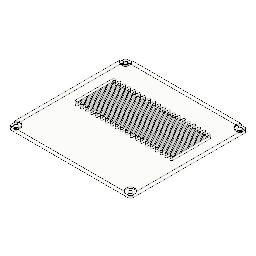
CaseLid v4 (Autodesk Fusion 360 design; units mm, degrees)
Autodesk Fusion 360 part; units mm, degrees
sketch "Sketch1" plane through (0, 0, 0) normal (0, 0, 1) x (1, 0, 0)
  line L0 (0, 0) -> (98, 0)
  line L1 (98, 0) -> (98, 94)
  line L2 (98, 94) -> (0, 94)
  line L3 (0, 94) -> (0, 0)
  dimension "d1" = 98
  dimension "d2" = 94
  constraint horizontal L0
  constraint vertical L1
  constraint horizontal L2
  constraint vertical L3
  constraint coincident L0.start L3.end
  measures "d1" distance of L0.start L0.end
  measures "d2" distance of L0.start L2.end
extrude "Extrude1" add sketch "Sketch1" along normal blind 3
fillet "Fillet1" radius 2 4 edges at (98, 0, 1.5) (98, 94, 1.5) (0, 94, 1.5) (0, 0, 1.5)
sketch "Sketch2" plane through (0, 0, 3) normal (0, 0, 1) x (-1, 0, 0)
  arc A0 (0, -2) -> (-2, 0) centre (-2, -2) ccw
  line L0 (-2, 0) -> (-96, 0)
  arc A1 (-96, 0) -> (-98, -2) centre (-96, -2) ccw
  line L1 (-98, -2) -> (-98, -92)
  arc A2 (-98, -92) -> (-96, -94) centre (-96, -92) ccw
  line L2 (-96, -94) -> (-2, -94)
  arc A3 (-2, -94) -> (0, -92) centre (-2, -92) ccw
  line L3 (0, -92) -> (0, -2)
  line L4 (-3, -91) -> (-95, -91) construction
  line L5 (-95, -91) -> (-95, -3) construction
  line L6 (-95, -3) -> (-3, -3) construction
  line L7 (-3, -3) -> (-3, -91) construction
  dimension "d6" = 92
  dimension "d7" = 88
  dimension "d8" = 3
  dimension "d9" = 3
  constraint horizontal L4
  constraint vertical L5
  constraint horizontal L6
  constraint vertical L7
  measures "d6" distance of L4.start L4.end
  measures "d7" distance of L4.start L6.end
  measures "d8" distance of L2 L4
  measures "d9" distance of L3 L7
hole "Hole1" at (3, 91, 3) at (95, 91, 3) at (95, 3, 3) at (3, 3, 3) direction (0, 0, -1) diameter 3 end through all counterbore diameter 7 counterbore depth 1
sketch "Sketch3" plane through (0, 0, 3) normal (0, 0, 1) x (-1, 0, 0)
  arc A0 (-98, -4.8028) -> (-93.1972, 0) centre (-95, -3) ccw
  line L0 (-98, -4.8028) -> (-98, -89.1972)
  arc A1 (-93.1972, -94) -> (-98, -89.1972) centre (-95, -91) ccw
  line L1 (-93.1972, -94) -> (-4.8028, -94)
  arc A2 (0, -89.1972) -> (-4.8028, -94) centre (-3, -91) ccw
  line L2 (0, -89.1972) -> (0, -4.8028)
  arc A3 (-4.8028, 0) -> (0, -4.8028) centre (-3, -3) ccw
  line L3 (-4.8028, 0) -> (-93.1972, 0)
  line L4 (-10, -74) -> (-10, -44)
  arc A4 (-10, -44) -> (-12, -44) centre (-11, -44) ccw
  line L5 (-12, -44) -> (-12, -74)
  arc A5 (-12, -74) -> (-10, -74) centre (-11, -74) ccw
  line L6 (-16, -44) -> (-16, -74)
  arc A6 (-14, -44) -> (-16, -44) centre (-15, -44) ccw
  line L7 (-14, -74) -> (-14, -44)
  arc A7 (-16, -74) -> (-14, -74) centre (-15, -74) ccw
  line L8 (-20, -44) -> (-20, -74)
  arc A8 (-18, -44) -> (-20, -44) centre (-19, -44) ccw
  line L9 (-18, -74) -> (-18, -44)
  arc A9 (-20, -74) -> (-18, -74) centre (-19, -74) ccw
  line L10 (-24, -44) -> (-24, -74)
  arc A10 (-22, -44) -> (-24, -44) centre (-23, -44) ccw
  line L11 (-22, -74) -> (-22, -44)
  arc A11 (-24, -74) -> (-22, -74) centre (-23, -74) ccw
  line L12 (-28, -44) -> (-28, -74)
  arc A12 (-26, -44) -> (-28, -44) centre (-27, -44) ccw
  line L13 (-26, -74) -> (-26, -44)
  arc A13 (-28, -74) -> (-26, -74) centre (-27, -74) ccw
  line L14 (-32, -44) -> (-32, -74)
  arc A14 (-30, -44) -> (-32, -44) centre (-31, -44) ccw
  line L15 (-30, -74) -> (-30, -44)
  arc A15 (-32, -74) -> (-30, -74) centre (-31, -74) ccw
  line L16 (-36, -44) -> (-36, -74)
  arc A16 (-34, -44) -> (-36, -44) centre (-35, -44) ccw
  line L17 (-34, -74) -> (-34, -44)
  arc A17 (-36, -74) -> (-34, -74) centre (-35, -74) ccw
  line L18 (-40, -44) -> (-40, -74)
  arc A18 (-38, -44) -> (-40, -44) centre (-39, -44) ccw
  line L19 (-38, -74) -> (-38, -44)
  arc A19 (-40, -74) -> (-38, -74) centre (-39, -74) ccw
  line L20 (-44, -44) -> (-44, -74)
  arc A20 (-42, -44) -> (-44, -44) centre (-43, -44) ccw
  line L21 (-42, -74) -> (-42, -44)
  arc A21 (-44, -74) -> (-42, -74) centre (-43, -74) ccw
  line L22 (-48, -44) -> (-48, -74)
  arc A22 (-46, -44) -> (-48, -44) centre (-47, -44) ccw
  line L23 (-46, -74) -> (-46, -44)
  arc A23 (-48, -74) -> (-46, -74) centre (-47, -74) ccw
  line L24 (-52, -44) -> (-52, -74)
  arc A24 (-50, -44) -> (-52, -44) centre (-51, -44) ccw
  line L25 (-50, -74) -> (-50, -44)
  arc A25 (-52, -74) -> (-50, -74) centre (-51, -74) ccw
  line L26 (-56, -44) -> (-56, -74)
  arc A26 (-54, -44) -> (-56, -44) centre (-55, -44) ccw
  line L27 (-54, -74) -> (-54, -44)
  arc A27 (-56, -74) -> (-54, -74) centre (-55, -74) ccw
  line L28 (-60, -44) -> (-60, -74)
  arc A28 (-58, -44) -> (-60, -44) centre (-59, -44) ccw
  line L29 (-58, -74) -> (-58, -44)
  arc A29 (-60, -74) -> (-58, -74) centre (-59, -74) ccw
  line L30 (-64, -44) -> (-64, -74)
  arc A30 (-62, -44) -> (-64, -44) centre (-63, -44) ccw
  line L31 (-62, -74) -> (-62, -44)
  arc A31 (-64, -74) -> (-62, -74) centre (-63, -74) ccw
  line L32 (-68, -44) -> (-68, -74)
  arc A32 (-66, -44) -> (-68, -44) centre (-67, -44) ccw
  line L33 (-66, -74) -> (-66, -44)
  arc A33 (-68, -74) -> (-66, -74) centre (-67, -74) ccw
  line L34 (-72, -44) -> (-72, -74)
  arc A34 (-70, -44) -> (-72, -44) centre (-71, -44) ccw
  line L35 (-70, -74) -> (-70, -44)
  arc A35 (-72, -74) -> (-70, -74) centre (-71, -74) ccw
  line L36 (-76, -44) -> (-76, -74)
  arc A36 (-74, -44) -> (-76, -44) centre (-75, -44) ccw
  line L37 (-74, -74) -> (-74, -44)
  arc A37 (-76, -74) -> (-74, -74) centre (-75, -74) ccw
  line L38 (-80, -44) -> (-80, -74)
  arc A38 (-78, -44) -> (-80, -44) centre (-79, -44) ccw
  line L39 (-78, -74) -> (-78, -44)
  arc A39 (-80, -74) -> (-78, -74) centre (-79, -74) ccw
  line L40 (-84, -44) -> (-84, -74)
  arc A40 (-82, -44) -> (-84, -44) centre (-83, -44) ccw
  line L41 (-82, -74) -> (-82, -44)
  arc A41 (-84, -74) -> (-82, -74) centre (-83, -74) ccw
  line L42 (-88, -44) -> (-88, -74)
  arc A42 (-86, -44) -> (-88, -44) centre (-87, -44) ccw
  line L43 (-86, -74) -> (-86, -44)
  arc A43 (-88, -74) -> (-86, -74) centre (-87, -74) ccw
  dimension "d15" = 2
  dimension "d16" = 30
  dimension "d17" = 20
  dimension "d20" = -4
  dimension "d21" = 0
  constraint vertical L4
  constraint tangent L4 A4
  constraint tangent A4 L5
  constraint parallel L4 L5
  constraint tangent L5 A5
  constraint tangent L4 A5
  measures "d15" distance of L4 L5
  measures "d16" distance of A4.centre A5.centre
  measures "d17" distance of L1 A5.centre
extrude "Extrude2" cut sketch "Sketch3" against normal through all contours L4 A4 L5 A5 | L6 A6 L7 A7 | L8 A8 L9 A9 | L10 A10 L11 A11 | L12 A12 L13 A13 | L14 A14 L15 A15 | L16 A16 L17 A17 | L18 A18 L19 A19 | L20 A20 L21 A21 | L22 A22 L23 A23 | L24 A24 L25 A25 | L26 A26 L27 A27 | L28 A28 L29 A29 | L30 A30 L31 A31 | L32 A32 L33 A33 | L34 A34 L35 A35 | L36 A36 L37 A37 | L38 A38 L39 A39 | L40 A40 L41 A41 | L42 A42 L43 A43
